Autodesk Fusion 360 part; units mm, degrees
(part 8 of 11)
  line L29 (-6.5693, -15.9779) -> (-6.6258, -16.0167)
  arc A59 (-6.9671, -15.9608) -> (-6.6258, -16.0167) centre (-6.7672, -15.8105) ccw
  arc A60 (-6.9671, -15.9608) -> (-7.0372, -15.8693) centre (-11.6741, -19.5) ccw
  arc A61 (-7.0029, -15.5252) -> (-7.0372, -15.8693) centre (-6.8404, -15.7152) ccw
  line L30 (-7.0029, -15.5252) -> (-6.9508, -15.4807)
  spline S30 degree 5 poles (-6.9508, -15.4807) (-6.9487, -15.4789) (-6.9446, -15.4753) (-6.9385, -15.4697) (-6.9307, -15.462) (-6.9213, -15.452) (-6.9121, -15.4417) (-6.9031, -15.4312) (-6.8942, -15.4206) (-6.8853, -15.4099) (-6.8765, -15.3992) (-6.8678, -15.3883) (-6.8592, -15.3774) (-6.8507, -15.3663) (-6.8424, -15.3551) (-6.8341, -15.3437) (-6.826, -15.3323) (-6.818, -15.3207) (-6.81, -15.3091) (-6.8021, -15.2974) (-6.7943, -15.2856) (-6.7865, -15.2737) (-6.7789, -15.2618) (-6.7713, -15.2498) (-6.7638, -15.2377) (-6.7564, -15.2255) (-6.749, -15.2132) (-6.7417, -15.2009) (-6.7345, -15.1885) (-6.7274, -15.176) (-6.7203, -15.1634) (-6.7134, -15.1508) (-6.7064, -15.1382) (-6.6996, -15.1254) (-6.6928, -15.1126) (-6.6861, -15.0997) (-6.6794, -15.0868) (-6.6728, -15.0738) (-6.6663, -15.0607) (-6.6598, -15.0476) (-6.6534, -15.0344) (-6.6471, -15.0212) (-6.6409, -15.0079) (-6.6347, -14.9946) (-6.6285, -14.9812) (-6.6224, -14.9677) (-6.6164, -14.9542) (-6.6105, -14.9406) (-6.6046, -14.927) (-6.5988, -14.9133) (-6.593, -14.8996) (-6.5873, -14.8858) (-6.5816, -14.872) (-6.576, -14.8581) (-6.5705, -14.8442) (-6.565, -14.8302) (-6.5596, -14.8161) (-6.5543, -14.8021) (-6.549, -14.7879) (-6.5438, -14.7737) (-6.5386, -14.7595) (-6.5335, -14.7452) (-6.5284, -14.7309) (-6.5234, -14.7166) (-6.5185, -14.7021) (-6.5136, -14.6877) (-6.5088, -14.6732) (-6.504, -14.6586) (-6.4993, -14.644) (-6.4947, -14.6294) (-6.4901, -14.6147) (-6.4865, -14.6029) (-6.4838, -14.5941) (-6.482, -14.5882) (-6.4811, -14.5852) knots 0 0 0 0 0 0 0.01428571 0.02857143 0.04285714 0.05714286 0.07142857 0.08571429 0.1 0.11428571 0.12857143 0.14285714 0.15714286 0.17142857 0.18571429 0.2 0.21428571 0.22857143 0.24285714 0.25714286 0.27142857 0.28571429 0.3 0.31428571 0.32857143 0.34285714 0.35714286 0.37142857 0.38571429 0.4 0.41428571 0.42857143 0.44285714 0.45714286 0.47142857 0.48571429 0.5 0.51428571 0.52857143 0.54285714 0.55714286 0.57142857 0.58571429 0.6 0.61428571 0.62857143 0.64285714 0.65714286 0.67142857 0.68571429 0.7 0.71428571 0.72857143 0.74285714 0.75714286 0.77142857 0.78571429 0.8 0.81428571 0.82857143 0.84285714 0.85714286 0.87142857 0.88571429 0.9 0.91428571 0.92857143 0.94285714 0.95714286 0.97142857 0.98571429 1 1 1 1 1 1
  arc A62 (-6.4811, -14.5852) -> (-6.7594, -14.307) centre (-11.6741, -19.5) ccw
  spline S31 degree 5 poles (-6.7594, -14.307) (-6.7623, -14.3079) (-6.7682, -14.3097) (-6.7771, -14.3123) (-6.7889, -14.316) (-6.8035, -14.3206) (-6.8182, -14.3252) (-6.8328, -14.3299) (-6.8473, -14.3347) (-6.8618, -14.3395) (-6.8763, -14.3444) (-6.8907, -14.3493) (-6.9051, -14.3543) (-6.9194, -14.3594) (-6.9337, -14.3645) (-6.9479, -14.3696) (-6.9621, -14.3749) (-6.9762, -14.3802) (-6.9903, -14.3855) (-7.0043, -14.3909) (-7.0183, -14.3964) (-7.0322, -14.4019) (-7.0461, -14.4075) (-7.0599, -14.4131) (-7.0737, -14.4188) (-7.0875, -14.4246) (-7.1011, -14.4304) (-7.1148, -14.4363) (-7.1283, -14.4423) (-7.1418, -14.4483) (-7.1553, -14.4544) (-7.1687, -14.4605) (-7.1821, -14.4667) (-7.1953, -14.473) (-7.2086, -14.4793) (-7.2218, -14.4857) (-7.2349, -14.4922) (-7.2479, -14.4987) (-7.2609, -14.5053) (-7.2739, -14.5119) (-7.2867, -14.5186) (-7.2995, -14.5254) (-7.3123, -14.5323) (-7.325, -14.5392) (-7.3376, -14.5462) (-7.3501, -14.5533) (-7.3626, -14.5604) (-7.375, -14.5676) (-7.3873, -14.5749) (-7.3996, -14.5822) (-7.4118, -14.5896) (-7.4239, -14.5971) (-7.4359, -14.6047) (-7.4479, -14.6124) (-7.4597, -14.6201) (-7.4715, -14.628) (-7.4832, -14.6359) (-7.4949, -14.6438) (-7.5064, -14.6519) (-7.5179, -14.66) (-7.5292, -14.6682) (-7.5404, -14.6766) (-7.5515, -14.6851) (-7.5625, -14.6937) (-7.5733, -14.7024) (-7.584, -14.7112) (-7.5947, -14.7201) (-7.6053, -14.729) (-7.6158, -14.738) (-7.6261, -14.7471) (-7.6361, -14.7566) (-7.6439, -14.7644) (-7.6494, -14.7705) (-7.6531, -14.7746) (-7.6548, -14.7767) knots -1 -1 -1 -1 -1 -1 -0.98571429 -0.97142857 -0.95714286 -0.94285714 -0.92857143 -0.91428571 -0.9 -0.88571429 -0.87142857 -0.85714286 -0.84285714 -0.82857143 -0.81428571 -0.8 -0.78571429 -0.77142857 -0.75714286 -0.74285714 -0.72857143 -0.71428571 -0.7 -0.68571429 -0.67142857 -0.65714286 -0.64285714 -0.62857143 -0.61428571 -0.6 -0.58571429 -0.57142857 -0.55714286 -0.54285714 -0.52857143 -0.51428571 -0.5 -0.48571429 -0.47142857 -0.45714286 -0.44285714 -0.42857143 -0.41428571 -0.4 -0.38571429 -0.37142857 -0.35714286 -0.34285714 -0.32857143 -0.31428571 -0.3 -0.28571429 -0.27142857 -0.25714286 -0.24285714 -0.22857143 -0.21428571 -0.2 -0.18571429 -0.17142857 -0.15714286 -0.14285714 -0.12857143 -0.11428571 -0.1 -0.08571429 -0.07142857 -0.05714286 -0.04285714 -0.02857143 -0.01428571 0 0 0 0 0 0
  line L31 (-7.6548, -14.7767) -> (-7.6994, -14.8287)
  arc A63 (-8.0435, -14.8631) -> (-7.6994, -14.8287) centre (-7.8894, -14.6662) ccw
  arc A64 (-8.0435, -14.8631) -> (-8.1349, -14.7929) centre (-11.6741, -19.5) ccw
  arc A65 (-8.1908, -14.4516) -> (-8.1349, -14.7929) centre (-7.9847, -14.5931) ccw
  line L32 (-8.1908, -14.4516) -> (-8.152, -14.3952)
  spline S32 degree 5 poles (-8.152, -14.3952) (-8.1505, -14.3929) (-8.1474, -14.3883) (-8.143, -14.3814) (-8.1374, -14.3719) (-8.1309, -14.3598) (-8.1247, -14.3475) (-8.1188, -14.335) (-8.1129, -14.3224) (-8.1071, -14.3098) (-8.1014, -14.2972) (-8.0958, -14.2845) (-8.0903, -14.2717) (-8.085, -14.2588) (-8.0798, -14.2458) (-8.0748, -14.2327) (-8.0699, -14.2195) (-8.0651, -14.2063) (-8.0604, -14.193) (-8.0558, -14.1796) (-8.0513, -14.1662) (-8.0469, -14.1527) (-8.0426, -14.1392) (-8.0384, -14.1256) (-8.0343, -14.112) (-8.0303, -14.0983) (-8.0263, -14.0846) (-8.0225, -14.0708) (-8.0188, -14.0569) (-8.0151, -14.043) (-8.0115, -14.0291) (-8.008, -14.0151) (-8.0046, -14.001) (-8.0013, -13.987) (-7.9981, -13.9728) (-7.9949, -13.9587) (-7.9918, -13.9444) (-7.9888, -13.9302) (-7.9859, -13.9159) (-7.9831, -13.9015) (-7.9803, -13.8872) (-7.9776, -13.8727) (-7.975, -13.8583) (-7.9725, -13.8438) (-7.97, -13.8292) (-7.9676, -13.8147) (-7.9653, -13.8) (-7.9631, -13.7854) (-7.9609, -13.7707) (-7.9588, -13.756) (-7.9568, -13.7412) (-7.9548, -13.7265) (-7.953, -13.7116) (-7.9512, -13.6968) (-7.9494, -13.6819) (-7.9478, -13.667) (-7.9462, -13.652) (-7.9447, -13.637) (-7.9432, -13.622) (-7.9418, -13.6069) (-7.9405, -13.5919) (-7.9393, -13.5768) (-7.9381, -13.5616) (-7.937, -13.5464) (-7.936, -13.5312) (-7.935, -13.516) (-7.9341, -13.5008) (-7.9333, -13.4855) (-7.9325, -13.4702) (-7.9318, -13.4548) (-7.9312, -13.4395) (-7.9307, -13.4271) (-7.9304, -13.4179) (-7.9302, -13.4117) (-7.9301, -13.4086) knots 0 0 0 0 0 0 0.01428571 0.02857143 0.04285714 0.05714286 0.07142857 0.08571429 0.1 0.11428571 0.12857143 0.14285714 0.15714286 0.17142857 0.18571429 0.2 0.21428571 0.22857143 0.24285714 0.25714286 0.27142857 0.28571429 0.3 0.31428571 0.32857143 0.34285714 0.35714286 0.37142857 0.38571429 0.4 0.41428571 0.42857143 0.44285714 0.45714286 0.47142857 0.48571429 0.5 0.51428571 0.52857143 0.54285714 0.55714286 0.57142857 0.58571429 0.6 0.61428571 0.62857143 0.64285714 0.65714286 0.67142857 0.68571429 0.7 0.71428571 0.72857143 0.74285714 0.75714286 0.77142857 0.78571429 0.8 0.81428571 0.82857143 0.84285714 0.85714286 0.87142857 0.88571429 0.9 0.91428571 0.92857143 0.94285714 0.95714286 0.97142857 0.98571429 1 1 1 1 1 1
  arc A66 (-7.9301, -13.4086) -> (-8.2709, -13.2119) centre (-11.6741, -19.5) ccw
  spline S33 degree 5 poles (-8.2709, -13.2119) (-8.2735, -13.2135) (-8.2788, -13.2168) (-8.2866, -13.2217) (-8.2971, -13.2282) (-8.31, -13.2364) (-8.323, -13.2447) (-8.3359, -13.253) (-8.3487, -13.2614) (-8.3614, -13.2698) (-8.3741, -13.2783) (-8.3868, -13.2868) (-8.3994, -13.2953) (-8.4119, -13.3039) (-8.4244, -13.3125) (-8.4368, -13.3212) (-8.4491, -13.3299) (-8.4614, -13.3387) (-8.4736, -13.3475) (-8.4858, -13.3564) (-8.4978, -13.3653) (-8.5099, -13.3742) (-8.5218, -13.3832) (-8.5337, -13.3922) (-8.5456, -13.4013) (-8.5573, -13.4104) (-8.569, -13.4196) (-8.5807, -13.4288) (-8.5923, -13.4381) (-8.6038, -13.4474) (-8.6152, -13.4567) (-8.6265, -13.4661) (-8.6378, -13.4756) (-8.649, -13.4851) (-8.6602, -13.4946) (-8.6713, -13.5042) (-8.6823, -13.5138) (-8.6932, -13.5235) (-8.704, -13.5332) (-8.7148, -13.543) (-8.7255, -13.5528) (-8.7361, -13.5627) (-8.7467, -13.5726) (-8.7571, -13.5826) (-8.7675, -13.5926) (-8.7778, -13.6027) (-8.788, -13.6128) (-8.7981, -13.623) (-8.8081, -13.6332) (-8.8181, -13.6435) (-8.8279, -13.6538) (-8.8377, -13.6642) (-8.8473, -13.6746) (-8.8569, -13.6851) (-8.8663, -13.6957) (-8.8757, -13.7063) (-8.885, -13.7169) (-8.8941, -13.7276) (-8.9032, -13.7384) (-8.9122, -13.7492) (-8.921, -13.7601) (-8.9297, -13.7711) (-8.9382, -13.7821) (-8.9465, -13.7933) (-8.9547, -13.8045) (-8.9628, -13.8158) (-8.9709, -13.8271) (-8.9788, -13.8384) (-8.9866, -13.8499) (-8.9942, -13.8614) (-9.0014, -13.8731) (-9.0069, -13.8826) (-9.0107, -13.8899) (-9.0131, -13.8949) (-9.0143, -13.8974) knots -1 -1 -1 -1 -1 -1 -0.98571429 -0.97142857 -0.95714286 -0.94285714 -0.92857143 -0.91428571 -0.9 -0.88571429 -0.87142857 -0.85714286 -0.84285714 -0.82857143 -0.81428571 -0.8 -0.78571429 -0.77142857 -0.75714286 -0.74285714 -0.72857143 -0.71428571 -0.7 -0.68571429 -0.67142857 -0.65714286 -0.64285714 -0.62857143 -0.61428571 -0.6 -0.58571429 -0.57142857 -0.55714286 -0.54285714 -0.52857143 -0.51428571 -0.5 -0.48571429 -0.47142857 -0.45714286 -0.44285714 -0.42857143 -0.41428571 -0.4 -0.38571429 -0.37142857 -0.35714286 -0.34285714 -0.32857143 -0.31428571 -0.3 -0.28571429 -0.27142857 -0.25714286 -0.24285714 -0.22857143 -0.21428571 -0.2 -0.18571429 -0.17142857 -0.15714286 -0.14285714 -0.12857143 -0.11428571 -0.1 -0.08571429 -0.07142857 -0.05714286 -0.04285714 -0.02857143 -0.01428571 0 0 0 0 0 0
  line L33 (-9.0143, -13.8974) -> (-9.0438, -13.9592)
  arc A67 (-9.3673, -14.0814) -> (-9.0438, -13.9592) centre (-9.2694, -13.8514) ccw
  arc A68 (-9.3673, -14.0814) -> (-9.4738, -14.0373) centre (-11.6741, -19.5) ccw
  arc A69 (-9.6161, -13.7221) -> (-9.4738, -14.0373) centre (-9.3804, -13.8054) ccw
  line L34 (-9.6161, -13.7221) -> (-9.5933, -13.6575)
  spline S34 degree 5 poles (-9.5933, -13.6575) (-9.5924, -13.6549) (-9.5906, -13.6497) (-9.5881, -13.6419) (-9.5852, -13.6313) (-9.5821, -13.6179) (-9.5793, -13.6044) (-9.5767, -13.5908) (-9.5743, -13.5771) (-9.572, -13.5635) (-9.5697, -13.5498) (-9.5676, -13.536) (-9.5656, -13.5222) (-9.5638, -13.5084) (-9.5622, -13.4945) (-9.5607, -13.4806) (-9.5594, -13.4666) (-9.5582, -13.4525) (-9.5571, -13.4385) (-9.5561, -13.4244) (-9.5553, -13.4103) (-9.5545, -13.3961) (-9.5538, -13.382) (-9.5533, -13.3678) (-9.5528, -13.3535) (-9.5525, -13.3393) (-9.5523, -13.325) (-9.5521, -13.3106) (-9.5521, -13.2963) (-9.5522, -13.2819) (-9.5523, -13.2675) (-9.5526, -13.2531) (-9.5529, -13.2387) (-9.5533, -13.2242) (-9.5539, -13.2097) (-9.5545, -13.1952) (-9.5552, -13.1807) (-9.556, -13.1661) (-9.5569, -13.1516) (-9.5578, -13.137) (-9.5589, -13.1224) (-9.56, -13.1077) (-9.5612, -13.0931) (-9.5625, -13.0784) (-9.5639, -13.0638) (-9.5654, -13.0491) (-9.5669, -13.0344) (-9.5686, -13.0196) (-9.5703, -13.0049) (-9.5721, -12.9901) (-9.5739, -12.9753) (-9.5759, -12.9606) (-9.5779, -12.9458) (-9.58, -12.9309) (-9.5822, -12.9161) (-9.5845, -12.9013) (-9.5868, -12.8864) (-9.5892, -12.8715) (-9.5917, -12.8567) (-9.5942, -12.8418) (-9.5969, -12.8269) (-9.5996, -12.8119) (-9.6024, -12.797) (-9.6052, -12.7821) (-9.6082, -12.7671) (-9.6112, -12.7522) (-9.6142, -12.7372) (-9.6174, -12.7222) (-9.6206, -12.7072) (-9.6239, -12.6922) (-9.6273, -12.6772) (-9.63, -12.6652) (-9.6321, -12.6562) (-9.6335, -12.6502) (-9.6342, -12.6472) knots 0 0 0 0 0 0 0.01428571 0.02857143 0.04285714 0.05714286 0.07142857 0.08571429 0.1 0.11428571 0.12857143 0.14285714 0.15714286 0.17142857 0.18571429 0.2 0.21428571 0.22857143 0.24285714 0.25714286 0.27142857 0.28571429 0.3 0.31428571 0.32857143 0.34285714 0.35714286 0.37142857 0.38571429 0.4 0.41428571 0.42857143 0.44285714 0.45714286 0.47142857 0.48571429 0.5 0.51428571 0.52857143 0.54285714 0.55714286 0.57142857 0.58571429 0.6 0.61428571 0.62857143 0.64285714 0.65714286 0.67142857 0.68571429 0.7 0.71428571 0.72857143 0.74285714 0.75714286 0.77142857 0.78571429 0.8 0.81428571 0.82857143 0.84285714 0.85714286 0.87142857 0.88571429 0.9 0.91428571 0.92857143 0.94285714 0.95714286 0.97142857 0.98571429 1 1 1 1 1 1
  arc A70 (-9.6342, -12.6472) -> (-10.0143, -12.5453) centre (-11.6741, -19.5) ccw
  spline S35 degree 5 poles (-10.0143, -12.5453) (-10.0164, -12.5476) (-10.0207, -12.5521) (-10.027, -12.5588) (-10.0354, -12.5679) (-10.0458, -12.5792) (-10.0562, -12.5905) (-10.0664, -12.6019) (-10.0767, -12.6133) (-10.0868, -12.6247) (-10.0969, -12.6362) (-10.1069, -12.6476) (-10.1168, -12.6592) (-10.1267, -12.6707) (-10.1365, -12.6823) (-10.1463, -12.6938) (-10.1559, -12.7055) (-10.1655, -12.7171) (-10.175, -12.7288) (-10.1845, -12.7405) (-10.1939, -12.7522) (-10.2032, -12.764) (-10.2124, -12.7757) (-10.2216, -12.7875) (-10.2306, -12.7994) (-10.2396, -12.8112) (-10.2486, -12.8231) (-10.2574, -12.835) (-10.2662, -12.847) (-10.2749, -12.8589) (-10.2835, -12.8709) (-10.2921, -12.883) (-10.3005, -12.895) (-10.3089, -12.9071) (-10.3172, -12.9192) (-10.3254, -12.9313) (-10.3335, -12.9435) (-10.3416, -12.9556) (-10.3496, -12.9678) (-10.3574, -12.9801) (-10.3652, -12.9923) (-10.3729, -13.0046) (-10.3805, -13.0169) (-10.388, -13.0292) (-10.3955, -13.0416) (-10.4028, -13.054) (-10.41, -13.0664) (-10.4172, -13.0789) (-10.4242, -13.0913) (-10.4312, -13.1038) (-10.438, -13.1163) (-10.4448, -13.1289) (-10.4514, -13.1415) (-10.4579, -13.1541) (-10.4643, -13.1667) (-10.4706, -13.1794) (-10.4768, -13.1921) (-10.4829, -13.2048) (-10.4888, -13.2175) (-10.4947, -13.2303) (-10.5004, -13.2431) (-10.5059, -13.256) (-10.5113, -13.2688) (-10.5165, -13.2818) (-10.5215, -13.2947) (-10.5264, -13.3077) (-10.5312, -13.3207) (-10.536, -13.3338) (-10.5405, -13.3468) (-10.5449, -13.3599) (-10.5488, -13.3731) (-10.5516, -13.3837) (-10.5534, -13.3917) (-10.5545, -13.3971) (-10.555, -13.3998) knots -1 -1 -1 -1 -1 -1 -0.98571429 -0.97142857 -0.95714286 -0.94285714 -0.92857143 -0.91428571 -0.9 -0.88571429 -0.87142857 -0.85714286 -0.84285714 -0.82857143 -0.81428571 -0.8 -0.78571429 -0.77142857 -0.75714286 -0.74285714 -0.72857143 -0.71428571 -0.7 -0.68571429 -0.67142857 -0.65714286 -0.64285714 -0.62857143 -0.61428571 -0.6 -0.58571429 -0.57142857 -0.55714286 -0.54285714 -0.52857143 -0.51428571 -0.5 -0.48571429 -0.47142857 -0.45714286 -0.44285714 -0.42857143 -0.41428571 -0.4 -0.38571429 -0.37142857 -0.35714286 -0.34285714 -0.32857143 -0.31428571 -0.3 -0.28571429 -0.27142857 -0.25714286 -0.24285714 -0.22857143 -0.21428571 -0.2 -0.18571429 -0.17142857 -0.15714286 -0.14285714 -0.12857143 -0.11428571 -0.1 -0.08571429 -0.07142857 -0.05714286 -0.04285714 -0.02857143 -0.01428571 0 0 0 0 0 0
  line L35 (-10.555, -13.3998) -> (-10.5675, -13.4672)
  arc A71 (-10.8484, -13.669) -> (-10.5675, -13.4672) centre (-10.8133, -13.4215) ccw
  arc A72 (-10.8484, -13.669) -> (-10.9626, -13.6539) centre (-11.6741, -19.5) ccw
  arc A73 (-11.1816, -13.3863) -> (-10.9626, -13.6539) centre (-10.9324, -13.4058) ccw
  line L36 (-11.1816, -13.3863) -> (-11.1763, -13.318)
  spline S36 degree 5 poles (-11.1763, -13.318) (-11.1761, -13.3153) (-11.1757, -13.3098) (-11.1754, -13.3016) (-11.1753, -13.2906) (-11.1757, -13.2768) (-11.1765, -13.2631) (-11.1776, -13.2493) (-11.1788, -13.2355) (-11.1801, -13.2217) (-11.1815, -13.2079) (-11.183, -13.194) (-11.1846, -13.1802) (-11.1864, -13.1664) (-11.1885, -13.1525) (-11.1907, -13.1387) (-11.193, -13.1248) (-11.1955, -13.111) (-11.1981, -13.0971) (-11.2008, -13.0832) (-11.2036, -13.0694) (-11.2065, -13.0555) (-11.2095, -13.0417) (-11.2127, -13.0278) (-11.2159, -13.0139) (-11.2193, -13.0001) (-11.2228, -12.9862) (-11.2264, -12.9723) (-11.23, -12.9585) (-11.2338, -12.9446) (-11.2377, -12.9307) (-11.2417, -12.9169) (-11.2457, -12.903) (-11.2499, -12.8891) (-11.2541, -12.8753) (-11.2585, -12.8614) (-11.2629, -12.8476) (-11.2675, -12.8337) (-11.2721, -12.8199) (-11.2768, -12.806) (-11.2816, -12.7922) (-11.2865, -12.7784) (-11.2915, -12.7645) (-11.2965, -12.7507) (-11.3016, -12.7369) (-11.3069, -12.7231) (-11.3122, -12.7093) (-11.3176, -12.6955) (-11.323, -12.6817) (-11.3286, -12.6679) (-11.3342, -12.6541) (-11.3399, -12.6403) (-11.3457, -12.6265) (-11.3516, -12.6128) (-11.3575, -12.599) (-11.3635, -12.5853) (-11.3696, -12.5715) (-11.3758, -12.5578) (-11.3821, -12.544) (-11.3884, -12.5303) (-11.3948, -12.5166) (-11.4013, -12.5029) (-11.4078, -12.4892) (-11.4145, -12.4755) (-11.4212, -12.4618) (-11.4279, -12.4481) (-11.4348, -12.4345) (-11.4417, -12.4208) (-11.4487, -12.4072) (-11.4558, -12.3936) (-11.4629, -12.3799) (-11.4687, -12.369) (-11.473, -12.3609) (-11.4759, -12.3554) (-11.4774, -12.3527) knots 0 0 0 0 0 0 0.01428571 0.02857143 0.04285714 0.05714286 0.07142857 0.08571429 0.1 0.11428571 0.12857143 0.14285714 0.15714286 0.17142857 0.18571429 0.2 0.21428571 0.22857143 0.24285714 0.25714286 0.27142857 0.28571429 0.3 0.31428571 0.32857143 0.34285714 0.35714286 0.37142857 0.38571429 0.4 0.41428571 0.42857143 0.44285714 0.45714286 0.47142857 0.48571429 0.5 0.51428571 0.52857143 0.54285714 0.55714286 0.57142857 0.58571429 0.6 0.61428571 0.62857143 0.64285714 0.65714286 0.67142857 0.68571429 0.7 0.71428571 0.72857143 0.74285714 0.75714286 0.77142857 0.78571429 0.8 0.81428571 0.82857143 0.84285714 0.85714286 0.87142857 0.88571429 0.9 0.91428571 0.92857143 0.94285714 0.95714286 0.97142857 0.98571429 1 1 1 1 1 1
  arc A74 (-11.4774, -12.3527) -> (-11.8709, -12.3527) centre (-11.6741, -19.5) ccw
  spline S37 degree 5 poles (-11.8709, -12.3527) (-11.8724, -12.3554) (-11.8753, -12.3609) (-11.8796, -12.369) (-11.8854, -12.3799) (-11.8925, -12.3936) (-11.8996, -12.4072) (-11.9066, -12.4208) (-11.9135, -12.4345) (-11.9203, -12.4481) (-11.9271, -12.4618) (-11.9338, -12.4755) (-11.9404, -12.4892) (-11.947, -12.5029) (-11.9535, -12.5166) (-11.9599, -12.5303) (-11.9662, -12.544) (-11.9725, -12.5578) (-11.9786, -12.5715) (-11.9847, -12.5853) (-11.9908, -12.599) (-11.9967, -12.6128) (-12.0026, -12.6265) (-12.0084, -12.6403) (-12.0141, -12.6541) (-12.0197, -12.6679) (-12.0253, -12.6817) (-12.0307, -12.6955) (-12.0361, -12.7093) (-12.0414, -12.7231) (-12.0466, -12.7369) (-12.0518, -12.7507) (-12.0568, -12.7645) (-12.0618, -12.7784) (-12.0667, -12.7922) (-12.0715, -12.806) (-12.0762, -12.8199) (-12.0808, -12.8337) (-12.0853, -12.8476) (-12.0898, -12.8614) (-12.0941, -12.8753) (-12.0984, -12.8891) (-12.1025, -12.903) (-12.1066, -12.9169) (-12.1106, -12.9307) (-12.1145, -12.9446) (-12.1182, -12.9585) (-12.1219, -12.9723) (-12.1255, -12.9862) (-12.129, -13.0001) (-12.1324, -13.0139) (-12.1356, -13.0278) (-12.1388, -13.0417) (-12.1418, -13.0555) (-12.1447, -13.0694) (-12.1475, -13.0832) (-12.1502, -13.0971) (-12.1528, -13.111) (-12.1553, -13.1248) (-12.1576, -13.1387) (-12.1598, -13.1525) (-12.1618, -13.1664) (-12.1637, -13.1802) (-12.1653, -13.194) (-12.1668, -13.2079) (-12.1682, -13.2217) (-12.1695, -13.2355) (-12.1707, -13.2493) (-12.1717, -13.2631) (-12.1725, -13.2768) (-12.173, -13.2906) (-12.1729, -13.3016) (-12.1725, -13.3098) (-12.1722, -13.3153) (-12.172, -13.318) knots -1 -1 -1 -1 -1 -1 -0.98571429 -0.97142857 -0.95714286 -0.94285714 -0.92857143 -0.91428571 -0.9 -0.88571429 -0.87142857 -0.85714286 -0.84285714 -0.82857143 -0.81428571 -0.8 -0.78571429 -0.77142857 -0.75714286 -0.74285714 -0.72857143 -0.71428571 -0.7 -0.68571429 -0.67142857 -0.65714286 -0.64285714 -0.62857143 -0.61428571 -0.6 -0.58571429 -0.57142857 -0.55714286 -0.54285714 -0.52857143 -0.51428571 -0.5 -0.48571429 -0.47142857 -0.45714286 -0.44285714 -0.42857143 -0.41428571 -0.4 -0.38571429 -0.37142857 -0.35714286 -0.34285714 -0.32857143 -0.31428571 -0.3 -0.28571429 -0.27142857 -0.25714286 -0.24285714 -0.22857143 -0.21428571 -0.2 -0.18571429 -0.17142857 -0.15714286 -0.14285714 -0.12857143 -0.11428571 -0.1 -0.08571429 -0.07142857 -0.05714286 -0.04285714 -0.02857143 -0.01428571 0 0 0 0 0 0
  line L37 (-12.172, -13.318) -> (-12.1666, -13.3863)
  arc A75 (-12.3857, -13.6539) -> (-12.1666, -13.3863) centre (-12.4159, -13.4058) ccw
  arc A76 (-12.3857, -13.6539) -> (-12.4999, -13.669) centre (-11.6741, -19.5) ccw
  arc A77 (-12.7808, -13.4672) -> (-12.4999, -13.669) centre (-12.535, -13.4215) ccw
  line L38 (-12.7808, -13.4672) -> (-12.7933, -13.3998)
  spline S38 degree 5 poles (-12.7933, -13.3998) (-12.7938, -13.3971) (-12.7949, -13.3917) (-12.7967, -13.3837) (-12.7994, -13.3731) (-12.8034, -13.3599) (-12.8077, -13.3468) (-12.8123, -13.3338) (-12.817, -13.3207) (-12.8219, -13.3077) (-12.8268, -13.2947) (-12.8318, -13.2818) (-12.837, -13.2688) (-12.8423, -13.256) (-12.8479, -13.2431) (-12.8536, -13.2303) (-12.8594, -13.2175) (-12.8654, -13.2048) (-12.8715, -13.1921) (-12.8777, -13.1794) (-12.884, -13.1667) (-12.8904, -13.1541) (-12.8969, -13.1415) (-12.9035, -13.1289) (-12.9103, -13.1163) (-12.9171, -13.1038) (-12.9241, -13.0913) (-12.9311, -13.0789) (-12.9382, -13.0664) (-12.9455, -13.054) (-12.9528, -13.0416) (-12.9602, -13.0292) (-12.9678, -13.0169) (-12.9754, -13.0046) (-12.9831, -12.9923) (-12.9908, -12.9801) (-12.9987, -12.9678) (-13.0067, -12.9556) (-13.0147, -12.9435) (-13.0229, -12.9313) (-13.0311, -12.9192) (-13.0394, -12.9071) (-13.0478, -12.895) (-13.0562, -12.883) (-13.0648, -12.8709) (-13.0734, -12.8589) (-13.0821, -12.847) (-13.0908, -12.835) (-13.0997, -12.8231) (-13.1086, -12.8112) (-13.1176, -12.7994) (-13.1267, -12.7875) (-13.1359, -12.7757) (-13.1451, -12.764) (-13.1544, -12.7522) (-13.1638, -12.7405) (-13.1732, -12.7288) (-13.1828, -12.7171) (-13.1924, -12.7055) (-13.202, -12.6938) (-13.2118, -12.6823) (-13.2216, -12.6707) (-13.2314, -12.6592) (-13.2414, -12.6476) (-13.2514, -12.6362) (-13.2615, -12.6247) (-13.2716, -12.6133) (-13.2818, -12.6019) (-13.2921, -12.5905) (-13.3025, -12.5792) (-13.3129, -12.5679) (-13.3213, -12.5588) (-13.3276, -12.5521) (-13.3318, -12.5476) (-13.3339, -12.5453) knots 0 0 0 0 0 0 0.01428571 0.02857143 0.04285714 0.05714286 0.07142857 0.08571429 0.1 0.11428571 0.12857143 0.14285714 0.15714286 0.17142857 0.18571429 0.2 0.21428571 0.22857143 0.24285714 0.25714286 0.27142857 0.28571429 0.3 0.31428571 0.32857143 0.34285714 0.35714286 0.37142857 0.38571429 0.4 0.41428571 0.42857143 0.44285714 0.45714286 0.47142857 0.48571429 0.5 0.51428571 0.52857143 0.54285714 0.55714286 0.57142857 0.58571429 0.6 0.61428571 0.62857143 0.64285714 0.65714286 0.67142857 0.68571429 0.7 0.71428571 0.72857143 0.74285714 0.75714286 0.77142857 0.78571429 0.8 0.81428571 0.82857143 0.84285714 0.85714286 0.87142857 0.88571429 0.9 0.91428571 0.92857143 0.94285714 0.95714286 0.97142857 0.98571429 1 1 1 1 1 1
  arc A78 (-13.3339, -12.5453) -> (-13.714, -12.6472) centre (-11.6741, -19.5) ccw
  spline S39 degree 5 poles (-13.714, -12.6472) (-13.7148, -12.6502) (-13.7162, -12.6562) (-13.7183, -12.6652) (-13.721, -12.6772) (-13.7244, -12.6922) (-13.7277, -12.7072) (-13.7309, -12.7222) (-13.734, -12.7372) (-13.7371, -12.7522) (-13.7401, -12.7671) (-13.743, -12.7821) (-13.7459, -12.797) (-13.7487, -12.8119) (-13.7514, -12.8269) (-13.754, -12.8418) (-13.7566, -12.8567) (-13.7591, -12.8715) (-13.7615, -12.8864) (-13.7638, -12.9013) (-13.7661, -12.9161) (-13.7683, -12.9309) (-13.7704, -12.9458) (-13.7724, -12.9606) (-13.7743, -12.9753) (-13.7762, -12.9901) (-13.778, -13.0049) (-13.7797, -13.0196) (-13.7813, -13.0344) (-13.7829, -13.0491) (-13.7844, -13.0638) (-13.7857, -13.0784) (-13.7871, -13.0931) (-13.7883, -13.1077) (-13.7894, -13.1224) (-13.7905, -13.137) (-13.7914, -13.1516) (-13.7923, -13.1661) (-13.7931, -13.1807) (-13.7938, -13.1952) (-13.7944, -13.2097) (-13.7949, -13.2242) (-13.7954, -13.2387) (-13.7957, -13.2531) (-13.796, -13.2675) (-13.7961, -13.2819) (-13.7962, -13.2963) (-13.7962, -13.3106) (-13.796, -13.325) (-13.7958, -13.3393) (-13.7955, -13.3535) (-13.795, -13.3678) (-13.7945, -13.382) (-13.7938, -13.3961) (-13.793, -13.4103) (-13.7921, -13.4244) (-13.7912, -13.4385) (-13.7901, -13.4525) (-13.7889, -13.4666) (-13.7876, -13.4806) (-13.7861, -13.4945) (-13.7845, -13.5084) (-13.7827, -13.5222) (-13.7807, -13.536) (-13.7786, -13.5498) (-13.7763, -13.5635) (-13.774, -13.5771) (-13.7716, -13.5908) (-13.769, -13.6044) (-13.7662, -13.6179) (-13.7631, -13.6313) (-13.7602, -13.6419) (-13.7577, -13.6497) (-13.7559, -13.6549) (-13.755, -13.6575) knots -1 -1 -1 -1 -1 -1 -0.98571429 -0.97142857 -0.95714286 -0.94285714 -0.92857143 -0.91428571 -0.9 -0.88571429 -0.87142857 -0.85714286 -0.84285714 -0.82857143 -0.81428571 -0.8 -0.78571429 -0.77142857 -0.75714286 -0.74285714 -0.72857143 -0.71428571 -0.7 -0.68571429 -0.67142857 -0.65714286 -0.64285714 -0.62857143 -0.61428571 -0.6 -0.58571429 -0.57142857 -0.55714286 -0.54285714 -0.52857143 -0.51428571 -0.5 -0.48571429 -0.47142857 -0.45714286 -0.44285714 -0.42857143 -0.41428571 -0.4 -0.38571429 -0.37142857 -0.35714286 -0.34285714 -0.32857143 -0.31428571 -0.3 -0.28571429 -0.27142857 -0.25714286 -0.24285714 -0.22857143 -0.21428571 -0.2 -0.18571429 -0.17142857 -0.15714286 -0.14285714 -0.12857143 -0.11428571 -0.1 -0.08571429 -0.07142857 -0.05714286 -0.04285714 -0.02857143 -0.01428571 0 0 0 0 0 0
  line L39 (-13.755, -13.6575) -> (-13.7322, -13.7221)
  arc A79 (-13.8745, -14.0373) -> (-13.7322, -13.7221) centre (-13.9679, -13.8054) ccw
  arc A80 (-13.8745, -14.0373) -> (-13.981, -14.0814) centre (-11.6741, -19.5) ccw
  arc A81 (-14.3045, -13.9592) -> (-13.981, -14.0814) centre (-14.0789, -13.8514) ccw
  line L40 (-14.3045, -13.9592) -> (-14.334, -13.8974)
  spline S40 degree 5 poles (-14.334, -13.8974) (-14.3352, -13.8949) (-14.3376, -13.8899) (-14.3414, -13.8826) (-14.3469, -13.8731) (-14.3541, -13.8614) (-14.3617, -13.8499) (-14.3695, -13.8384) (-14.3774, -13.8271) (-14.3854, -13.8158) (-14.3935, -13.8045) (-14.4017, -13.7933) (-14.4101, -13.7821) (-14.4186, -13.7711) (-14.4273, -13.7601) (-14.4361, -13.7492) (-14.4451, -13.7384) (-14.4541, -13.7276) (-14.4633, -13.7169) (-14.4726, -13.7063) (-14.4819, -13.6957) (-14.4914, -13.6851) (-14.5009, -13.6746) (-14.5106, -13.6642) (-14.5204, -13.6538) (-14.5302, -13.6435) (-14.5402, -13.6332) (-14.5502, -13.623) (-14.5603, -13.6128) (-14.5705, -13.6027) (-14.5808, -13.5926) (-14.5912, -13.5826) (-14.6016, -13.5726) (-14.6122, -13.5627) (-14.6228, -13.5528) (-14.6335, -13.543) (-14.6442, -13.5332) (-14.6551, -13.5235) (-14.666, -13.5138) (-14.677, -13.5042) (-14.6881, -13.4946) (-14.6992, -13.4851) (-14.7104, -13.4756) (-14.7217, -13.4661) (-14.7331, -13.4567) (-14.7445, -13.4474) (-14.756, -13.4381) (-14.7676, -13.4288) (-14.7792, -13.4196) (-14.7909, -13.4104) (-14.8027, -13.4013) (-14.8145, -13.3922) (-14.8264, -13.3832) (-14.8384, -13.3742) (-14.8504, -13.3653) (-14.8625, -13.3564) (-14.8747, -13.3475) (-14.8869, -13.3387) (-14.8992, -13.3299) (-14.9115, -13.3212) (-14.9239, -13.3125) (-14.9364, -13.3039) (-14.9489, -13.2953) (-14.9615, -13.2868) (-14.9741, -13.2783) (-14.9868, -13.2698) (-14.9996, -13.2614) (-15.0124, -13.253) (-15.0253, -13.2447) (-15.0382, -13.2364) (-15.0512, -13.2282) (-15.0617, -13.2217) (-15.0695, -13.2168) (-15.0748, -13.2135) (-15.0774, -13.2119) knots 0 0 0 0 0 0 0.01428571 0.02857143 0.04285714 0.05714286 0.07142857 0.08571429 0.1 0.11428571 0.12857143 0.14285714 0.15714286 0.17142857 0.18571429 0.2 0.21428571 0.22857143 0.24285714 0.25714286 0.27142857 0.28571429 0.3 0.31428571 0.32857143 0.34285714 0.35714286 0.37142857 0.38571429 0.4 0.41428571 0.42857143 0.44285714 0.45714286 0.47142857 0.48571429 0.5 0.51428571 0.52857143 0.54285714 0.55714286 0.57142857 0.58571429 0.6 0.61428571 0.62857143 0.64285714 0.65714286 0.67142857 0.68571429 0.7 0.71428571 0.72857143 0.74285714 0.75714286 0.77142857 0.78571429 0.8 0.81428571 0.82857143 0.84285714 0.85714286 0.87142857 0.88571429 0.9 0.91428571 0.92857143 0.94285714 0.95714286 0.97142857 0.98571429 1 1 1 1 1 1
  arc A82 (-15.0774, -13.2119) -> (-15.4182, -13.4086) centre (-11.6741, -19.5) ccw
  spline S41 degree 5 poles (-15.4182, -13.4086) (-15.4181, -13.4117) (-15.4179, -13.4179) (-15.4176, -13.4271) (-15.4171, -13.4395) (-15.4165, -13.4548) (-15.4158, -13.4702) (-15.415, -13.4855) (-15.4142, -13.5008) (-15.4133, -13.516) (-15.4123, -13.5312) (-15.4113, -13.5464) (-15.4102, -13.5616) (-15.409, -13.5768) (-15.4078, -13.5919) (-15.4064, -13.6069) (-15.4051, -13.622) (-15.4036, -13.637) (-15.4021, -13.652) (-15.4005, -13.667) (-15.3988, -13.6819) (-15.3971, -13.6968) (-15.3953, -13.7116) (-15.3934, -13.7265) (-15.3915, -13.7412) (-15.3895, -13.756) (-15.3874, -13.7707) (-15.3852, -13.7854) (-15.383, -13.8) (-15.3807, -13.8147) (-15.3783, -13.8292) (-15.3758, -13.8438) (-15.3733, -13.8583) (-15.3707, -13.8727) (-15.368, -13.8872) (-15.3652, -13.9015) (-15.3624, -13.9159) (-15.3595, -13.9302) (-15.3565, -13.9444) (-15.3534, -13.9587) (-15.3502, -13.9728) (-15.347, -13.987) (-15.3437, -14.001) (-15.3402, -14.0151) (-15.3368, -14.0291) (-15.3332, -14.043) (-15.3295, -14.0569) (-15.3258, -14.0708) (-15.3219, -14.0846) (-15.318, -14.0983) (-15.314, -14.112) (-15.3099, -14.1256) (-15.3057, -14.1392) (-15.3014, -14.1527) (-15.297, -14.1662) (-15.2924, -14.1796) (-15.2879, -14.193) (-15.2832, -14.2063) (-15.2784, -14.2195) (-15.2735, -14.2327) (-15.2685, -14.2458) (-15.2633, -14.2588) (-15.258, -14.2717) (-15.2525, -14.2845) (-15.2469, -14.2972) (-15.2412, -14.3098) (-15.2354, -14.3224) (-15.2295, -14.335) (-15.2235, -14.3475) (-15.2173, -14.3598) (-15.2108, -14.3719) (-15.2053, -14.3814) (-15.2009, -14.3883) (-15.1978, -14.3929) (-15.1962, -14.3952) knots -1 -1 -1 -1 -1 -1 -0.98571429 -0.97142857 -0.95714286 -0.94285714 -0.92857143 -0.91428571 -0.9 -0.88571429 -0.87142857 -0.85714286 -0.84285714 -0.82857143 -0.81428571 -0.8 -0.78571429 -0.77142857 -0.75714286 -0.74285714 -0.72857143 -0.71428571 -0.7 -0.68571429 -0.67142857 -0.65714286 -0.64285714 -0.62857143 -0.61428571 -0.6 -0.58571429 -0.57142857 -0.55714286 -0.54285714 -0.52857143 -0.51428571 -0.5 -0.48571429 -0.47142857 -0.45714286 -0.44285714 -0.42857143 -0.41428571 -0.4 -0.38571429 -0.37142857 -0.35714286 -0.34285714 -0.32857143 -0.31428571 -0.3 -0.28571429 -0.27142857 -0.25714286 -0.24285714 -0.22857143 -0.21428571 -0.2 -0.18571429 -0.17142857 -0.15714286 -0.14285714 -0.12857143 -0.11428571 -0.1 -0.08571429 -0.07142857 -0.05714286 -0.04285714 -0.02857143 -0.01428571 0 0 0 0 0 0
  line L41 (-15.1962, -14.3952) -> (-15.1575, -14.4516)
  arc A83 (-15.2134, -14.7929) -> (-15.1575, -14.4516) centre (-15.3636, -14.5931) ccw
  arc A84 (-15.2134, -14.7929) -> (-15.3048, -14.8631) centre (-11.6741, -19.5) ccw
  arc A85 (-15.6489, -14.8287) -> (-15.3048, -14.8631) centre (-15.4589, -14.6662) ccw
  line L42 (-15.6489, -14.8287) -> (-15.6934, -14.7767)
  spline S42 degree 5 poles (-15.6934, -14.7767) (-15.6952, -14.7746) (-15.6988, -14.7705) (-15.7044, -14.7644) (-15.7121, -14.7566) (-15.7222, -14.7471) (-15.7325, -14.738) (-15.743, -14.729) (-15.7536, -14.7201) (-15.7642, -14.7112) (-15.775, -14.7024) (-15.7858, -14.6937) (-15.7968, -14.6851) (-15.8078, -14.6766) (-15.8191, -14.6682) (-15.8304, -14.66) (-15.8419, -14.6519) (-15.8534, -14.6438) (-15.8651, -14.6359) (-15.8768, -14.628) (-15.8885, -14.6201) (-15.9004, -14.6124) (-15.9123, -14.6047) (-15.9244, -14.5971) (-15.9365, -14.5896) (-15.9487, -14.5822) (-15.9609, -14.5749) (-15.9733, -14.5676) (-15.9857, -14.5604) (-15.9982, -14.5533) (-16.0107, -14.5462) (-16.0233, -14.5392) (-16.036, -14.5323) (-16.0487, -14.5254) (-16.0615, -14.5186) (-16.0744, -14.5119) (-16.0873, -14.5053) (-16.1003, -14.4987) (-16.1134, -14.4922) (-16.1265, -14.4857) (-16.1397, -14.4793) (-16.1529, -14.473) (-16.1662, -14.4667) (-16.1796, -14.4605) (-16.193, -14.4544) (-16.2064, -14.4483) (-16.22, -14.4423) (-16.2335, -14.4363) (-16.2471, -14.4304) (-16.2608, -14.4246) (-16.2746, -14.4188) (-16.2883, -14.4131) (-16.3022, -14.4075) (-16.3161, -14.4019) (-16.33, -14.3964) (-16.344, -14.3909) (-16.358, -14.3855) (-16.3721, -14.3802) (-16.3862, -14.3749) (-16.4004, -14.3696) (-16.4146, -14.3645) (-16.4289, -14.3594) (-16.4432, -14.3543) (-16.4576, -14.3493) (-16.472, -14.3444) (-16.4865, -14.3395) (-16.501, -14.3347) (-16.5155, -14.3299) (-16.5301, -14.3252) (-16.5447, -14.3206) (-16.5594, -14.316) (-16.5712, -14.3123) (-16.58, -14.3097) (-16.586, -14.3079) (-16.5889, -14.307) knots 0 0 0 0 0 0 0.01428571 0.02857143 0.04285714 0.05714286 0.07142857 0.08571429 0.1 0.11428571 0.12857143 0.14285714 0.15714286 0.17142857 0.18571429 0.2 0.21428571 0.22857143 0.24285714 0.25714286 0.27142857 0.28571429 0.3 0.31428571 0.32857143 0.34285714 0.35714286 0.37142857 0.38571429 0.4 0.41428571 0.42857143 0.44285714 0.45714286 0.47142857 0.48571429 0.5 0.51428571 0.52857143 0.54285714 0.55714286 0.57142857 0.58571429 0.6 0.61428571 0.62857143 0.64285714 0.65714286 0.67142857 0.68571429 0.7 0.71428571 0.72857143 0.74285714 0.75714286 0.77142857 0.78571429 0.8 0.81428571 0.82857143 0.84285714 0.85714286 0.87142857 0.88571429 0.9 0.91428571 0.92857143 0.94285714 0.95714286 0.97142857 0.98571429 1 1 1 1 1 1
  arc A86 (-16.5889, -14.307) -> (-16.8672, -14.5852) centre (-11.6741, -19.5) ccw
  spline S43 degree 5 poles (-16.8672, -14.5852) (-16.8663, -14.5882) (-16.8645, -14.5941) (-16.8618, -14.6029) (-16.8582, -14.6147) (-16.8536, -14.6294) (-16.8489, -14.644) (-16.8442, -14.6586) (-16.8395, -14.6732) (-16.8346, -14.6877) (-16.8298, -14.7021) (-16.8248, -14.7166) (-16.8198, -14.7309) (-16.8148, -14.7452) (-16.8097, -14.7595) (-16.8045, -14.7737) (-16.7993, -14.7879) (-16.794, -14.8021) (-16.7886, -14.8161) (-16.7832, -14.8302) (-16.7778, -14.8442) (-16.7722, -14.8581) (-16.7666, -14.872) (-16.761, -14.8858) (-16.7553, -14.8996) (-16.7495, -14.9133) (-16.7437, -14.927) (-16.7378, -14.9406) (-16.7319, -14.9542) (-16.7258, -14.9677) (-16.7198, -14.9812) (-16.7136, -14.9946) (-16.7074, -15.0079) (-16.7012, -15.0212) (-16.6948, -15.0344) (-16.6884, -15.0476) (-16.682, -15.0607) (-16.6755, -15.0738) (-16.6689, -15.0868) (-16.6622, -15.0997) (-16.6555, -15.1126) (-16.6487, -15.1254) (-16.6419, -15.1382) (-16.6349, -15.1508) (-16.6279, -15.1634) (-16.6209, -15.176) (-16.6137, -15.1885) (-16.6065, -15.2009) (-16.5993, -15.2132) (-16.5919, -15.2255) (-16.5845, -15.2377) (-16.577, -15.2498) (-16.5694, -15.2618) (-16.5617, -15.2737) (-16.554, -15.2856) (-16.5462, -15.2974) (-16.5383, -15.3091) (-16.5303, -15.3207) (-16.5223, -15.3323) (-16.5141, -15.3437) (-16.5059, -15.3551) (-16.4975, -15.3663) (-16.4891, -15.3774) (-16.4805, -15.3883) (-16.4717, -15.3992) (-16.4629, -15.4099) (-16.4541, -15.4206) (-16.4452, -15.4312) (-16.4362, -15.4417) (-16.427, -15.452) (-16.4176, -15.462) (-16.4097, -15.4697) (-16.4037, -15.4753) (-16.3995, -15.4789) (-16.3975, -15.4807) knots -1 -1 -1 -1 -1 -1 -0.98571429 -0.97142857 -0.95714286 -0.94285714 -0.92857143 -0.91428571 -0.9 -0.88571429 -0.87142857 -0.85714286 -0.84285714 -0.82857143 -0.81428571 -0.8 -0.78571429 -0.77142857 -0.75714286 -0.74285714 -0.72857143 -0.71428571 -0.7 -0.68571429 -0.67142857 -0.65714286 -0.64285714 -0.62857143 -0.61428571 -0.6 -0.58571429 -0.57142857 -0.55714286 -0.54285714 -0.52857143 -0.51428571 -0.5 -0.48571429 -0.47142857 -0.45714286 -0.44285714 -0.42857143 -0.41428571 -0.4 -0.38571429 -0.37142857 -0.35714286 -0.34285714 -0.32857143 -0.31428571 -0.3 -0.28571429 -0.27142857 -0.25714286 -0.24285714 -0.22857143 -0.21428571 -0.2 -0.18571429 -0.17142857 -0.15714286 -0.14285714 -0.12857143 -0.11428571 -0.1 -0.08571429 -0.07142857 -0.05714286 -0.04285714 -0.02857143 -0.01428571 0 0 0 0 0 0
  line L43 (-16.3975, -15.4807) -> (-16.3454, -15.5252)
  arc A87 (-16.3111, -15.8693) -> (-16.3454, -15.5252) centre (-16.5079, -15.7152) ccw
  arc A88 (-16.3111, -15.8693) -> (-16.3812, -15.9608) centre (-11.6741, -19.5) ccw
  arc A89 (-16.7225, -16.0167) -> (-16.3812, -15.9608) centre (-16.581, -15.8105) ccw
  line L44 (-16.7225, -16.0167) -> (-16.779, -15.9779)
  spline S44 degree 5 poles (-16.779, -15.9779) (-16.7812, -15.9763) (-16.7858, -15.9733) (-16.7928, -15.9689) (-16.8022, -15.9633) (-16.8144, -15.9568) (-16.8267, -15.9506) (-16.8391, -15.9446) (-16.8517, -15.9388) (-16.8643, -15.933) (-16.877, -15.9272) (-16.8897, -15.9216) (-16.9025, -15.9162) (-16.9154, -15.9108) (-16.9284, -15.9057) (-16.9415, -15.9006) (-16.9546, -15.8957) (-16.9679, -15.891) (-16.9812, -15.8863) (-16.9945, -15.8817) (-17.0079, -15.8772) (-17.0214, -15.8728) (-17.0349, -15.8685) (-17.0485, -15.8642) (-17.0621, -15.8601) (-17.0758, -15.8561) (-17.0896, -15.8522) (-17.1034, -15.8484) (-17.1172, -15.8446) (-17.1311, -15.841) (-17.1451, -15.8374) (-17.1591, -15.8339) (-17.1731, -15.8305) (-17.1872, -15.8272) (-17.2013, -15.8239) (-17.2155, -15.8208) (-17.2297, -15.8177) (-17.244, -15.8147) (-17.2583, -15.8118) (-17.2726, -15.8089) (-17.287, -15.8062) (-17.3014, -15.8035) (-17.3159, -15.8009) (-17.3304, -15.7983) (-17.3449, -15.7959) (-17.3595, -15.7935) (-17.3741, -15.7912) (-17.3887, -15.7889) (-17.4034, -15.7868) (-17.4181, -15.7847) (-17.4329, -15.7827) (-17.4477, -15.7807) (-17.4625, -15.7788) (-17.4774, -15.777) (-17.4923, -15.7753) (-17.5072, -15.7736) (-17.5221, -15.772) (-17.5371, -15.7705) (-17.5521, -15.7691) (-17.5672, -15.7677) (-17.5823, -15.7664) (-17.5974, -15.7651) (-17.6125, -15.764) (-17.6277, -15.7629) (-17.6429, -15.7618) (-17.6581, -15.7609) (-17.6734, -15.76) (-17.6887, -15.7591) (-17.704, -15.7583) (-17.7193, -15.7576) (-17.7347, -15.757) (-17.747, -15.7566) (-17.7562, -15.7562) (-17.7624, -15.7561) (-17.7655, -15.756) knots 0 0 0 0 0 0 0.01428571 0.02857143 0.04285714 0.05714286 0.07142857 0.08571429 0.1 0.11428571 0.12857143 0.14285714 0.15714286 0.17142857 0.18571429 0.2 0.21428571 0.22857143 0.24285714 0.25714286 0.27142857 0.28571429 0.3 0.31428571 0.32857143 0.34285714 0.35714286 0.37142857 0.38571429 0.4 0.41428571 0.42857143 0.44285714 0.45714286 0.47142857 0.48571429 0.5 0.51428571 0.52857143 0.54285714 0.55714286 0.57142857 0.58571429 0.6 0.61428571 0.62857143 0.64285714 0.65714286 0.67142857 0.68571429 0.7 0.71428571 0.72857143 0.74285714 0.75714286 0.77142857 0.78571429 0.8 0.81428571 0.82857143 0.84285714 0.85714286 0.87142857 0.88571429 0.9 0.91428571 0.92857143 0.94285714 0.95714286 0.97142857 0.98571429 1 1 1 1 1 1
  arc A90 (-17.7655, -15.756) -> (-17.9623, -16.0967) centre (-11.6741, -19.5) ccw
  spline S45 degree 5 poles (-17.9623, -16.0967) (-17.9606, -16.0994) (-17.9574, -16.1046) (-17.9525, -16.1125) (-17.9459, -16.1229) (-17.9377, -16.1359) (-17.9294, -16.1488) (-17.9211, -16.1617) (-17.9127, -16.1745) (-17.9043, -16.1873) (-17.8959, -16.2) (-17.8874, -16.2126) (-17.8788, -16.2252) (-17.8702, -16.2378) (-17.8616, -16.2502) (-17.8529, -16.2626) (-17.8442, -16.275) (-17.8354, -16.2872) (-17.8266, -16.2995) (-17.8178, -16.3116) (-17.8089, -16.3237) (-17.7999, -16.3357) (-17.7909, -16.3477) (-17.7819, -16.3596) (-17.7728, -16.3714) (-17.7637, -16.3832) (-17.7545, -16.3949) (-17.7453, -16.4065) (-17.7361, -16.4181) (-17.7268, -16.4296) (-17.7174, -16.441) (-17.708, -16.4524) (-17.6986, -16.4637) (-17.6891, -16.4749) (-17.6795, -16.4861) (-17.6699, -16.4971) (-17.6603, -16.5081) (-17.6506, -16.5191) (-17.6409, -16.5299) (-17.6311, -16.5407) (-17.6213, -16.5514) (-17.6114, -16.562) (-17.6015, -16.5725) (-17.5915, -16.583) (-17.5815, -16.5933) (-17.5715, -16.6036) (-17.5613, -16.6138) (-17.5512, -16.624) (-17.5409, -16.634) (-17.5307, -16.6439) (-17.5204, -16.6538) (-17.51, -16.6635) (-17.4995, -16.6732) (-17.489, -16.6827) (-17.4785, -16.6922) (-17.4679, -16.7016) (-17.4572, -16.7108) (-17.4465, -16.72) (-17.4358, -16.7291) (-17.4249, -16.738) (-17.4141, -16.7469) (-17.4031, -16.7555) (-17.392, -16.764) (-17.3809, -16.7724) (-17.3696, -16.7806) (-17.3584, -16.7887) (-17.347, -16.7967) (-17.3357, -16.8047) (-17.3243, -16.8125) (-17.3127, -16.82) (-17.301, -16.8273) (-17.2915, -16.8327) (-17.2842, -16.8365) (-17.2793, -16.839) (-17.2768, -16.8401) knots -1 -1 -1 -1 -1 -1 -0.98571429 -0.97142857 -0.95714286 -0.94285714 -0.92857143 -0.91428571 -0.9 -0.88571429 -0.87142857 -0.85714286 -0.84285714 -0.82857143 -0.81428571 -0.8 -0.78571429 -0.77142857 -0.75714286 -0.74285714 -0.72857143 -0.71428571 -0.7 -0.68571429 -0.67142857 -0.65714286 -0.64285714 -0.62857143 -0.61428571 -0.6 -0.58571429 -0.57142857 -0.55714286 -0.54285714 -0.52857143 -0.51428571 -0.5 -0.48571429 -0.47142857 -0.45714286 -0.44285714 -0.42857143 -0.41428571 -0.4 -0.38571429 -0.37142857 -0.35714286 -0.34285714 -0.32857143 -0.31428571 -0.3 -0.28571429 -0.27142857 -0.25714286 -0.24285714 -0.22857143 -0.21428571 -0.2 -0.18571429 -0.17142857 -0.15714286 -0.14285714 -0.12857143 -0.11428571 -0.1 -0.08571429 -0.07142857 -0.05714286 -0.04285714 -0.02857143 -0.01428571 0 0 0 0 0 0
  line L45 (-17.2768, -16.8401) -> (-17.215, -16.8697)
  arc A91 (-17.0927, -17.1932) -> (-17.215, -16.8697) centre (-17.3228, -17.0952) ccw
  arc A92 (-17.0927, -17.1932) -> (-17.1368, -17.2996) centre (-11.6741, -19.5) ccw
  arc A93 (-17.452, -17.442) -> (-17.1368, -17.2996) centre (-17.3687, -17.2062) ccw
  line L46 (-17.452, -17.442) -> (-17.5166, -17.4191)
  spline S46 degree 5 poles (-17.5166, -17.4191) (-17.5192, -17.4182) (-17.5244, -17.4165) (-17.5323, -17.414) (-17.5429, -17.4111) (-17.5563, -17.4079) (-17.5698, -17.4051) (-17.5834, -17.4026) (-17.597, -17.4002) (-17.6107, -17.3978) (-17.6244, -17.3956) (-17.6381, -17.3934) (-17.6519, -17.3915) (-17.6657, -17.3897) (-17.6796, -17.388) (-17.6936, -17.3866) (-17.7076, -17.3853) (-17.7216, -17.3841) (-17.7356, -17.383) (-17.7497, -17.382) (-17.7638, -17.3811) (-17.778, -17.3803) (-17.7922, -17.3797) (-17.8064, -17.3791) (-17.8206, -17.3787) (-17.8349, -17.3783) (-17.8492, -17.3781) (-17.8635, -17.378) (-17.8778, -17.378) (-17.8922, -17.378) (-17.9066, -17.3782) (-17.921, -17.3784) (-17.9355, -17.3788) (-17.9499, -17.3792) (-17.9644, -17.3797) (-17.9789, -17.3803) (-17.9935, -17.381) (-18.008, -17.3818) (-18.0226, -17.3827) (-18.0372, -17.3837) (-18.0518, -17.3847) (-18.0664, -17.3859) (-18.081, -17.3871) (-18.0957, -17.3884) (-18.1104, -17.3898) (-18.1251, -17.3912) (-18.1398, -17.3928) (-18.1545, -17.3944) (-18.1693, -17.3961) (-18.184, -17.3979) (-18.1988, -17.3998) (-18.2136, -17.4017) (-18.2284, -17.4038) (-18.2432, -17.4059) (-18.258, -17.4081) (-18.2729, -17.4103) (-18.2877, -17.4126) (-18.3026, -17.4151) (-18.3175, -17.4175) (-18.3324, -17.4201) (-18.3473, -17.4227) (-18.3622, -17.4255) (-18.3771, -17.4282) (-18.3921, -17.4311) (-18.407, -17.434) (-18.422, -17.437) (-18.437, -17.4401) (-18.4519, -17.4433) (-18.4669, -17.4465) (-18.4819, -17.4498) (-18.4969, -17.4531) (-18.5089, -17.4559) (-18.518, -17.458) (-18.524, -17.4594) (-18.527, -17.4601) knots 0 0 0 0 0 0 0.01428571 0.02857143 0.04285714 0.05714286 0.07142857 0.08571429 0.1 0.11428571 0.12857143 0.14285714 0.15714286 0.17142857 0.18571429 0.2 0.21428571 0.22857143 0.24285714 0.25714286 0.27142857 0.28571429 0.3 0.31428571 0.32857143 0.34285714 0.35714286 0.37142857 0.38571429 0.4 0.41428571 0.42857143 0.44285714 0.45714286 0.47142857 0.48571429 0.5 0.51428571 0.52857143 0.54285714 0.55714286 0.57142857 0.58571429 0.6 0.61428571 0.62857143 0.64285714 0.65714286 0.67142857 0.68571429 0.7 0.71428571 0.72857143 0.74285714 0.75714286 0.77142857 0.78571429 0.8 0.81428571 0.82857143 0.84285714 0.85714286 0.87142857 0.88571429 0.9 0.91428571 0.92857143 0.94285714 0.95714286 0.97142857 0.98571429 1 1 1 1 1 1
  arc A94 (-18.527, -17.4601) -> (-18.6288, -17.8402) centre (-11.6741, -19.5) ccw
  spline S47 degree 5 poles (-18.6288, -17.8402) (-18.6266, -17.8423) (-18.6221, -17.8465) (-18.6153, -17.8529) (-18.6063, -17.8612) (-18.595, -17.8717) (-18.5836, -17.882) (-18.5723, -17.8923) (-18.5609, -17.9025) (-18.5494, -17.9127) (-18.538, -17.9227) (-18.5265, -17.9328) (-18.515, -17.9427) (-18.5034, -17.9526) (-18.4919, -17.9624) (-18.4803, -17.9721) (-18.4687, -17.9818) (-18.457, -17.9914) (-18.4454, -18.0009) (-18.4337, -18.0104) (-18.4219, -18.0197) (-18.4102, -18.029) (-18.3984, -18.0383) (-18.3866, -18.0474) (-18.3748, -18.0565) (-18.3629, -18.0655) (-18.351, -18.0744) (-18.3391, -18.0833) (-18.3272, -18.0921) (-18.3152, -18.1008) (-18.3032, -18.1094) (-18.2912, -18.1179) (-18.2791, -18.1264) (-18.2671, -18.1348) (-18.255, -18.1431) (-18.2428, -18.1513) (-18.2307, -18.1594) (-18.2185, -18.1675) (-18.2063, -18.1754) (-18.1941, -18.1833) (-18.1818, -18.1911) (-18.1695, -18.1988) (-18.1572, -18.2064) (-18.1449, -18.2139) (-18.1325, -18.2213) (-18.1201, -18.2287) (-18.1077, -18.2359) (-18.0953, -18.243) (-18.0828, -18.2501) (-18.0703, -18.257) (-18.0578, -18.2639) (-18.0453, -18.2706) (-18.0327, -18.2772) (-18.0201, -18.2838) (-18.0074, -18.2901) (-17.9948, -18.2964) (-17.9821, -18.3026) (-17.9694, -18.3087) (-17.9566, -18.3147) (-17.9438, -18.3206) (-17.931, -18.3263) (-17.9182, -18.3318) (-17.9053, -18.3372) (-17.8924, -18.3423) (-17.8794, -18.3474) (-17.8664, -18.3523) (-17.8534, -18.3571) (-17.8404, -18.3618) (-17.8273, -18.3664) (-17.8142, -18.3707) (-17.8011, -18.3747) (-17.7904, -18.3775) (-17.7824, -18.3793) (-17.777, -18.3803) (-17.7743, -18.3808) knots -1 -1 -1 -1 -1 -1 -0.98571429 -0.97142857 -0.95714286 -0.94285714 -0.92857143 -0.91428571 -0.9 -0.88571429 -0.87142857 -0.85714286 -0.84285714 -0.82857143 -0.81428571 -0.8 -0.78571429 -0.77142857 -0.75714286 -0.74285714 -0.72857143 -0.71428571 -0.7 -0.68571429 -0.67142857 -0.65714286 -0.64285714 -0.62857143 -0.61428571 -0.6 -0.58571429 -0.57142857 -0.55714286 -0.54285714 -0.52857143 -0.51428571 -0.5 -0.48571429 -0.47142857 -0.45714286 -0.44285714 -0.42857143 -0.41428571 -0.4 -0.38571429 -0.37142857 -0.35714286 -0.34285714 -0.32857143 -0.31428571 -0.3 -0.28571429 -0.27142857 -0.25714286 -0.24285714 -0.22857143 -0.21428571 -0.2 -0.18571429 -0.17142857 -0.15714286 -0.14285714 -0.12857143 -0.11428571 -0.1 -0.08571429 -0.07142857 -0.05714286 -0.04285714 -0.02857143 -0.01428571 0 0 0 0 0 0
  line L47 (-17.7743, -18.3808) -> (-17.707, -18.3934)
  arc A95 (-17.5052, -18.6742) -> (-17.707, -18.3934) centre (-17.7527, -18.6392) ccw
  circle A96 centre (-11.6741, -19.5) radius 1.25
  circle A97 centre (-13, -17) radius 0.9
  circle A98 centre (1.6741, -19.5) radius 1.225
  circle A99 centre (-11.6741, -19.5) radius 1.225
  line L48 (-10, -5) -> (-10, -10)
  line L49 (-10, -10) -> (-18.1241, -19.7489)
  arc A100 (-18.1241, -19.7489) -> (-17.2201, -22.9266) centre (-16.5876, -21.0293) ccw
  line L50 (-17.2201, -22.9266) -> (-11.2199, -25.4807)
  arc A101 (-11.2199, -25.4807) -> (-8.6741, -26) centre (-8.6741, -19.5) ccw
  line L51 (-8.6741, -26) -> (-1.3259, -26)
  arc A102 (-1.3259, -26) -> (1.2199, -25.4807) centre (-1.3259, -19.5) ccw
  line L52 (1.2199, -25.4807) -> (7.2201, -22.9266)
  arc A103 (7.2201, -22.9266) -> (8.1241, -19.7489) centre (6.5876, -21.0293) ccw
  line L53 (8.1241, -19.7489) -> (0, -10)
  line L54 (0, -10) -> (0, -5)
  line L55 (0, -5) -> (-10, -5)
  arc A104 (-4.1569, -18.6742) -> (-4.1719, -18.7885) centre (1.6741, -19.5) ccw
  arc A105 (-4.4395, -19.0075) -> (-4.1719, -18.7885) centre (-4.4201, -18.7583) ccw
  line L56 (-4.4395, -19.0075) -> (-4.5078, -19.0022)
  spline S48 degree 5 poles (-4.5078, -19.0022) (-4.5106, -19.002) (-4.516, -19.0016) (-4.5243, -19.0013) (-4.5353, -19.0012) (-4.549, -19.0016) (-4.5628, -19.0024) (-4.5766, -19.0035) (-4.5904, -19.0046) (-4.6042, -19.0059) (-4.618, -19.0073) (-4.6318, -19.0088) (-4.6457, -19.0105) (-4.6595, -19.0123) (-4.6733, -19.0143) (-4.6872, -19.0165) (-4.701, -19.0189) (-4.7149, -19.0214) (-4.7288, -19.024) (-4.7426, -19.0267) (-4.7565, -19.0295) (-4.7703, -19.0324) (-4.7842, -19.0354) (-4.7981, -19.0385) (-4.8119, -19.0418) (-4.8258, -19.0452) (-4.8397, -19.0486) (-4.8535, -19.0522) (-4.8674, -19.0559) (-4.8813, -19.0597) (-4.8951, -19.0636) (-4.909, -19.0675) (-4.9229, -19.0716) (-4.9367, -19.0758) (-4.9506, -19.08) (-4.9644, -19.0844) (-4.9783, -19.0888) (-4.9921, -19.0933) (-5.006, -19.098) (-5.0198, -19.1027) (-5.0337, -19.1075) (-5.0475, -19.1123) (-5.0613, -19.1173) (-5.0751, -19.1224) (-5.089, -19.1275) (-5.1028, -19.1327) (-5.1166, -19.138) (-5.1304, -19.1434) (-5.1442, -19.1489) (-5.158, -19.1544) (-5.1718, -19.1601) (-5.1855, -19.1658) (-5.1993, -19.1716) (-5.2131, -19.1774) (-5.2269, -19.1834) (-5.2406, -19.1894) (-5.2544, -19.1955) (-5.2681, -19.2017) (-5.2818, -19.2079) (-5.2955, -19.2143) (-5.3093, -19.2207) (-5.323, -19.2271) (-5.3367, -19.2337) (-5.3504, -19.2403) (-5.364, -19.247) (-5.3777, -19.2538) (-5.3914, -19.2606) (-5.405, -19.2676) (-5.4187, -19.2746) (-5.4323, -19.2816) (-5.4459, -19.2887) (-5.4568, -19.2945) (-5.465, -19.2989) (-5.4704, -19.3018) (-5.4732, -19.3032) knots 0 0 0 0 0 0 0.01428571 0.02857143 0.04285714 0.05714286 0.07142857 0.08571429 0.1 0.11428571 0.12857143 0.14285714 0.15714286 0.17142857 0.18571429 0.2 0.21428571 0.22857143 0.24285714 0.25714286 0.27142857 0.28571429 0.3 0.31428571 0.32857143 0.34285714 0.35714286 0.37142857 0.38571429 0.4 0.41428571 0.42857143 0.44285714 0.45714286 0.47142857 0.48571429 0.5 0.51428571 0.52857143 0.54285714 0.55714286 0.57142857 0.58571429 0.6 0.61428571 0.62857143 0.64285714 0.65714286 0.67142857 0.68571429 0.7 0.71428571 0.72857143 0.74285714 0.75714286 0.77142857 0.78571429 0.8 0.81428571 0.82857143 0.84285714 0.85714286 0.87142857 0.88571429 0.9 0.91428571 0.92857143 0.94285714 0.95714286 0.97142857 0.98571429 1 1 1 1 1 1
  arc A106 (-5.4732, -19.3032) -> (-5.4732, -19.6968) centre (1.6741, -19.5) ccw